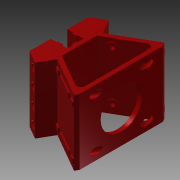
# Autodesk Inventor part: lower corner
Saved by Autodesk Inventor 2015 SP1 (Build 190203100, 203)
## iProperties
Created: 2015-01-28
Part Number: lower corner
Material: Generic
Document SubType Name: Modeling
Designer: Joseph
Density: 1 g/cm^3
Appearance: Red
Author: Joseph
Autodesk Inventor part; units mm, degrees
note: some values were not read from the file. Chosen so that the rebuilt part matches the saved one: direction of "Hole8".
sketch "Sketch1" plane through (0, 0, 0) normal (0, 0, 1) x (1, 0, 0)
  line L0 (7.9588, 40.9294) -> (17.9588, 23.6089)
  line L1 (17.9588, 23.6089) -> (65.5902, 51.1089)
  line L2 (7.9588, -48.8207) -> (17.9588, -31.5002)
  line L3 (17.9588, -31.5002) -> (65.5902, -59.0002)
  line L4 (65.5902, -59.0002) -> (68.0902, -54.6701)
  line L5 (65.5902, 51.1089) -> (68.0902, 46.7788)
  line L6 (17.039, 17.3044) -> (17.039, -25.1956)
  line L7 (-7.6578, 31.9131) -> (7.9588, 40.9294)
  line L8 (7.9588, -48.8207) -> (-7.6578, -39.8044)
  line L9 (63.0902, 43.892) -> (63.0902, -51.7833)
  line L10 (68.0902, 46.7788) -> (68.0902, -54.6701)
  line L11 (63.0902, 43.892) -> (17.039, 17.3044)
  line L12 (63.0902, -51.7833) -> (17.039, -25.1956)
  line L13 (63.0902, -12.2336) -> (68.0902, -12.2336) construction
  line L14 (63.0902, -51.7833) -> (60.5902, -56.1134) construction
  line L15 (63.0902, 43.892) -> (60.5902, 48.2222) construction
  line L16 (17.039, -3.9456) -> (63.0902, -3.9456) construction
  line L17 (-7.6578, 6.0639) -> (-7.6578, -13.9552) construction
  line L18 (-7.6578, 31.9131) -> (-7.6578, 6.0639)
  line L19 (-7.6578, -13.9552) -> (-7.6578, -39.8044)
  line L20 (-7.6578, -13.9552) -> (-0.4078, -13.9552)
  line L21 (5.0922, -13.9361) -> (12.3422, -13.9361)
  line L22 (12.3422, 6.0639) -> (5.0922, 6.0639)
  line L23 (-0.4078, 6.0639) -> (-7.6578, 6.0639)
  line L24 (12.3422, -6.6861) -> (10.8613, -6.6861)
  line L25 (10.8613, -6.6861) -> (10.8613, -1.1861)
  line L26 (10.8613, -1.1861) -> (12.3422, -1.1861)
  line L27 (5.0922, 6.0639) -> (5.0922, 4.5831)
  line L28 (5.0922, 4.5831) -> (-0.4078, 4.5831)
  line L29 (-0.4078, 4.5831) -> (-0.4078, 6.0639)
  line L30 (-0.4078, -13.9552) -> (-0.4078, -12.4552)
  line L31 (-0.4078, -12.4552) -> (5.0922, -12.4552)
  line L32 (5.0922, -12.4552) -> (5.0922, -13.9361)
  line L33 (12.3422, -13.9361) -> (12.3422, -6.6861)
  line L34 (12.3422, -1.1861) -> (12.3422, 6.0639)
  dimension "d11" = 20
  dimension "d12" = 55
  dimension "d110" = 42.5
  dimension "d176" = 5
  dimension "d177" = 60
  dimension "d178" = 120
  dimension "d179" = 60
  dimension "d181" = 20
  dimension "d184" = 1.5
  dimension "d185" = 5.5
  dimension "d186" = 20
  dimension "d195" = 34.8655
  dimension "d209" = 55
  constraints: 70 end point, 19 perpendicular, 15 equal length, 12 parallel, 6 point on line, 2 horizontal, 2 midpoint
  measures "d11" distance of L2.start L2.end
  measures "d12" distance of L2.end L3.end
  measures "d110" distance of L6.start L6.end
  measures "d176" distance of L3.end L4.end
  measures "d177" angle of L11 L12
  measures "d178" angle of L6 L12
  measures "d179" angle of L1 L3
  measures "d181" distance of L22.start L21.end
  measures "d184" distance of L20.end L30.end
  measures "d185" distance of L30.end L31.end
  measures "d186" distance between parallel lines of L17 L33
  measures "d195" distance from line of L0.start L22
  measures "d209" distance of L0.end L1.end
extrude "Extrusion13" add sketch "Sketch1" along normal blind 80
fillet "Fillet5" radius 5 2 edges at (63.0902, -51.7833, 40) (63.0902, 43.892, 40)
sketch "Sketch2" plane through (7.9588, 40.9294, 80) normal (0.8660254, 0.5, 0) x (0, 0, -1)
  line L0 (20, -20) -> (0, -20) construction
  circle A0 centre (10, -10) radius 10 construction
  circle A1 centre (70, -10) radius 10 construction
  line L1 (7, -21) -> (13, -21)
  line L2 (13, -21) -> (13, -19)
  line L3 (13, -19) -> (7, -19)
  line L4 (7, -19) -> (7, -21)
  line L5 (7, -21) -> (13, -19) construction
  line L6 (13, -21) -> (7, -19) construction
  line L7 (73, -21) -> (67, -21)
  line L8 (67, -21) -> (67, -19)
  line L9 (67, -19) -> (73, -19)
  line L10 (73, -19) -> (73, -21)
  line L11 (73, -21) -> (67, -19) construction
  line L12 (67, -21) -> (73, -19) construction
  line L13 (80, 0) -> (80, -20) projected
  line L14 (0, -20) -> (0, 0) projected
  line L15 (80, -20) -> (0, -20) projected
  line L16 (13, -19) -> (67, -19) construction
  point P0 (60, -34.2995)
  point P1 (10, -20)
  point P2 (70, -20)
  dimension "d11" = 20
  dimension "d168" = 20
  dimension "d19" = 20
  dimension "d23" = 6
  dimension "d24" = 2
  dimension "d25" = 6
  dimension "d26" = 2
  constraints: 28 end point, 5 horizontal, 4 midpoint, 4 parallel, 3 perpendicular, 2 vertical, 2 vertical alignment, 4 other
  measures "d19" distance of L0.start L0.end
  measures "d23" distance of L3.end L2.end
  measures "d24" distance of L2.end L1.end
  measures "d25" distance of L8.end L9.end
  measures "d26" distance of L7.end L8.end
extrude "Extrusion2" add sketch "Sketch2" along normal up to surface (55 mm away) from surface at 0
sketch "Sketch8" plane through (17.9588, -31.5002, 80) normal (0.8660254, -0.5, 0) x (0, 0, -1)
  line L0 (0, 0) -> (20, 0) construction
  line L1 (80, 0) -> (60, 0) construction
  line L2 (60, 0) -> (0, 0)
  line L3 (20, 0) -> (0, 0) construction
  line L4 (40, 0) -> (60, 0) construction
  line L5 (80, 0) -> (80, -20) projected
  circle A0 centre (70, -10) radius 10 construction
  line L6 (80, 0) -> (0, 0) projected
  line L7 (70, 0) -> (70, -20) construction
  line L8 (80, -20) -> (0, -20) construction
  line L9 (40, -20) -> (40, 0) construction
  line L10 (72.75, 1.5) -> (67.25, 1.5)
  line L11 (67.25, 1.5) -> (67.25, -1.5)
  line L12 (67.25, -1.5) -> (72.75, -1.5)
  line L13 (72.75, -1.5) -> (72.75, 1.5)
  line L14 (72.75, 1.5) -> (67.25, -1.5) construction
  line L15 (67.25, 1.5) -> (72.75, -1.5) construction
  line L16 (10, 0) -> (10, -20) construction
  line L17 (7.25, -1.5) -> (12.75, -1.5)
  line L18 (12.75, -1.5) -> (12.75, 1.5)
  line L19 (12.75, 1.5) -> (7.25, 1.5)
  line L20 (7.25, 1.5) -> (7.25, -1.5)
  line L21 (7.25, -1.5) -> (12.75, 1.5) construction
  line L22 (12.75, -1.5) -> (7.25, 1.5) construction
  point P0 (60, 16.0535)
  point P1 (60, 3.2816)
  dimension "d169" = 20
  dimension "d171" = 5.5
  dimension "d172" = 3
  dimension "d173" = 5.5
  dimension "d174" = 3
  constraints: 40 end point, 6 midpoint, 4 horizontal, 4 parallel, 2 perpendicular, 2 point on circle, 2 symmetric about line, 2 tangent, 1 centre point, 1 line through centre, 1 point on line, 1 vertical
  measures "d169" diameter of A0
  measures "d171" distance of L12.end L11.end
  measures "d172" distance of L11.end L10.end
  measures "d173" distance of L19.end L18.end
  measures "d174" distance of L18.end L17.end
extrude "Extrusion7" add sketch "Sketch8" along normal up to surface (55 mm away) from surface at 0
ref_plane "Work Plane20" through (33.539, 3.3832, 80) normal (0.5, 0.8660254, 0) x (0.8660254, -0.5, 0)
sketch "Sketch9" plane through (33.539, 3.3832, 80) normal (0.5, 0.8660254, 0) x (0.8660254, -0.5, 0)
  line L0 (58.9488, 70) -> (1.9893, 70) construction
  line L1 (48.9488, 10) -> (13.9488, 10) construction
  line L2 (13.9488, 10) -> (13.9488, 70) construction
  line L3 (13.9488, 70) -> (48.9488, 70) construction
  line L4 (48.9488, 70) -> (48.9488, 10) construction
  line L5 (58.9488, 72.75) -> (58.9488, 67.25) construction
  line L6 (58.9488, 12.75) -> (58.9488, 7.25) construction
  line L7 (48.9488, 10) -> (58.9488, 10) construction
  point P0 (-26.8584, -7)
  dimension "d73" = 35
  dimension "d205" = 10
  constraints: 12 end point, 4 coincident, 2 horizontal, 2 midpoint, 2 parallel, 1 collinear, 1 perpendicular, 1 point on line
  measures "d73" distance of L1.end L7.start
  measures "d205" distance of L7.start L7.end
hole "Hole2" at (75.93, -21.0912, 70) at (45.6191, -3.5912, 70) at (75.93, -21.0912, 10) at (45.6191, -3.5912, 10) direction (-0.5, -0.8660254, 0) diameter 4.5 end through all counterbore diameter 8 counterbore depth 32 clearance for "Socket Head Cap Screw" size "M4" standard "Ansi Metric M Profile"
ref_plane "Work Plane21" through (33.539, -11.2745, 0) normal (0.5, -0.8660254, 0) x (0.8660254, 0.5, 0)
sketch "Sketch10" plane through (33.539, -11.2745, 0) normal (0.5, -0.8660254, 0) x (0.8660254, 0.5, 0)
  line L0 (48.9488, 70) -> (13.9488, 70) construction
  line L1 (13.9488, 70) -> (13.9488, 10) construction
  line L2 (13.9488, 10) -> (48.9488, 10) construction
  line L3 (48.9488, 10) -> (48.9488, 70) construction
  line L4 (58.9488, 13) -> (58.9488, 7) construction
  line L5 (58.9488, 73) -> (58.9488, 67) construction
  line L6 (48.9488, 10) -> (58.9488, 10) construction
  line L7 (48.9488, 70) -> (58.9488, 70) construction
  point P0 (-25.1395, 13)
  dimension "d74" = 35
  dimension "d208" = 10
  constraints: 12 end point, 4 coincident, 2 collinear, 2 midpoint, 2 parallel, 1 horizontal, 1 perpendicular
  measures "d74" distance of L2.end L1.end
  measures "d208" distance between parallel lines of L3 L4
hole "Hole3" at (75.93, 13.1999, 70) at (75.93, 13.1999, 10) at (45.6191, -4.3001, 10) at (45.6191, -4.3001, 70) direction (-0.5, 0.8660254, 0) diameter 4.5 end through all counterbore diameter 8 counterbore depth 32 clearance for "Socket Head Cap Screw" size "M4" standard "Ansi Metric M Profile"
ref_plane "Work Plane18" through (7.9588, 40.9294, 0) normal (0, -1, 0) x (1, 0, 0)
sketch "Sketch20" plane through (7.9588, 40.9294, 0) normal (0, -1, 0) x (1, 0, 0)
  line L0 (-2.8667, 0) -> (-8.3667, 0) construction
  line L1 (-8.3667, 80) -> (-2.8667, 80) construction
  line L2 (-5.6167, 0) -> (-5.6167, 80) construction
  circle A0 centre (-5.6167, 70) radius 10
  circle A1 centre (-5.6167, 10) radius 10
  circle A2 centre (-5.6167, 40) radius 10
  point P0 (-7.9588, 0)
  point P1 (-5.6167, 30)
  point P2 (-5.6167, 50)
  dimension "d210" = 20
  dimension "d211" = 20
  dimension "d212" = 20
  constraints: 4 point on line, 3 centre point, 3 midpoint, 2 end point, 2 point on circle, 2 tangent
  measures "d210" diameter of A0
  measures "d211" diameter of A1
  measures "d212" diameter of A2
hole "Hole7" at (2.3422, 40.9294, 30) at (2.3422, 40.9294, 50) at (2.3422, 40.9294, 70) at (2.3422, 40.9294, 10) direction (0, -1, 0) diameter 4.5 end up to surface counterbore diameter 8 counterbore depth 16.35 clearance for "Socket Head Cap Screw" size "M4" standard "Ansi Metric M Profile"
ref_plane "Work Plane19" through (7.9588, -48.8207, 0) normal (0, -1, 0) x (1, 0, 0)
sketch "Sketch21" plane through (7.9588, -48.8207, 0) normal (0, -1, 0) x (1, 0, 0)
  line L0 (-8.3667, 0) -> (-2.8667, 0) projected
  line L1 (-2.8667, 80) -> (-8.3667, 80) projected
  line L2 (-5.6167, 80) -> (-5.6167, 0) construction
  circle A0 centre (-5.6167, 40) radius 10 construction
  circle A1 centre (-5.6167, 10) radius 10
  circle A2 centre (-5.6167, 70) radius 10
  point P0 (-7.9588, 0)
  point P1 (-5.6167, 50)
  point P2 (-5.6167, 30)
  point P3 (-5.6167, 70.2671)
  dimension "d196" = 20
  dimension "d213" = 20
  dimension "d214" = 20
  constraints: 4 point on line, 3 centre point, 3 midpoint, 2 end point, 2 point on circle, 2 tangent, 1 coincident
  measures "d196" diameter of A0
  measures "d213" diameter of A1
  measures "d214" diameter of A2
hole "Hole8" at (2.3422, -48.8207, 50) at (2.3422, -48.8207, 30) at (2.3422, -48.8207, 70.2671) at (2.3422, -48.8207, 10) direction (0, 1, 0) diameter 4.5 end up to surface counterbore diameter 8 counterbore depth 16.35 clearance for "Socket Head Cap Screw" size "M4" standard "Ansi Metric M Profile"
sketch "Sketch22" plane through (68.0902, -54.6701, 0) normal (1, 0, 0) x (0, 0, -1)
  circle A0 centre (-40, 50.7244) radius 25
  point P0 (0, 54.6701)
  dimension "d215" = 50
  constraints: 1 centre point
  measures "d215" diameter of A0
extrude "Extrusion14" cut sketch "Sketch22" against normal up to surface (5 mm away)
sketch "Sketch23" plane through (17.039, -25.1956, 0) normal (1, 0, 0) x (0, 0, -1)
  line L0 (0, 42.5) -> (0, 0) projected
  circle A0 centre (0, 21.25) radius 7.5
  point P0 (0, 25.1956)
  dimension "d218" = 15
  constraints: 1 centre point, 1 midpoint
  measures "d218" diameter of A0
extrude "Extrusion15" cut sketch "Sketch23" against normal up to surface (6.1777 mm away)
fillet "Fillet6" radius 2 4 edges at (17.039, -25.1956, 40) (17.039, 17.3044, 40) (68.0902, -54.6701, 40) (68.0902, 46.7788, 40)
sketch "Sketch24" plane through (55.5902, 39.5619, 0) normal (0.5, -0.8660254, 0) x (0.8660254, 0.5, 0)
  circle A0 centre (-30.5662, 70) radius 2.25 projected
  circle A1 centre (-30.5662, 10) radius 2.25 projected
  circle A2 centre (-30.5662, 70) radius 6
  circle A3 centre (-30.5662, 10) radius 6
  circle A4 centre (4.4338, 70) radius 2.25 projected
  circle A5 centre (4.4338, 10) radius 2.25 projected
  circle A6 centre (4.4338, 70) radius 6
  circle A7 centre (4.4338, 10) radius 6
  point P0 (-67.9235, 0)
  dimension "d222" = 12
  dimension "d223" = 12
  dimension "d228" = 12
  dimension "d229" = 12
  constraints: 4 centre point, 4 coincident
  measures "d222" diameter of A2
  measures "d223" diameter of A3
  measures "d228" diameter of A6
  measures "d229" diameter of A7
extrude "Extrusion16" add sketch "Sketch24" along normal blind 1
sketch "Sketch26" plane through (55.5902, -47.4532, 80) normal (0.5, 0.8660254, 0) x (0.8660254, -0.5, 0)
  circle A0 centre (-30.5662, 10) radius 2.25 projected
  circle A1 centre (-30.5662, 70) radius 2.25 projected
  circle A2 centre (4.4338, 10) radius 2.25 projected
  circle A3 centre (4.4338, 70) radius 2.25 projected
  circle A4 centre (-30.5662, 10) radius 6
  circle A5 centre (-30.5662, 70) radius 6
  circle A6 centre (4.4338, 70) radius 6
  circle A7 centre (4.4338, 10) radius 6
  point P0 (-71.8691, 80)
  dimension "d230" = 12
  dimension "d231" = 12
  dimension "d232" = 12
  dimension "d233" = 12
  constraints: 4 centre point, 4 coincident
  measures "d230" diameter of A4
  measures "d231" diameter of A5
  measures "d232" diameter of A6
  measures "d233" diameter of A7
extrude "Extrusion17" add sketch "Sketch26" along normal blind 1
sketch "Sketch27" plane through (17.2088, -32.7992, 67.25) normal (-0.5, -0.8660254, 0) x (0.8660254, -0.5, 0)
  circle A0 centre (45, 2.75) radius 2.25 projected
  circle A1 centre (10, 2.75) radius 2.25 projected
  circle A2 centre (10, -57.25) radius 2.25 projected
  circle A3 centre (45, -57.25) radius 2.25 projected
  line L0 (6.875, -60.375) -> (13.125, -60.375)
  line L1 (13.125, -60.375) -> (13.125, -54.125)
  line L2 (13.125, -54.125) -> (6.875, -54.125)
  line L3 (6.875, -54.125) -> (6.875, -60.375)
  line L4 (6.875, -60.375) -> (13.125, -54.125) construction
  line L5 (13.125, -60.375) -> (6.875, -54.125) construction
  line L6 (41.875, -60.375) -> (48.125, -60.375)
  line L7 (48.125, -60.375) -> (48.125, -54.125)
  line L8 (48.125, -54.125) -> (41.875, -54.125)
  line L9 (41.875, -54.125) -> (41.875, -60.375)
  line L10 (41.875, -60.375) -> (48.125, -54.125) construction
  line L11 (48.125, -60.375) -> (41.875, -54.125) construction
  line L12 (41.875, -0.375) -> (48.125, -0.375)
  line L13 (48.125, -0.375) -> (48.125, 5.875)
  line L14 (48.125, 5.875) -> (41.875, 5.875)
  line L15 (41.875, 5.875) -> (41.875, -0.375)
  line L16 (41.875, -0.375) -> (48.125, 5.875) construction
  line L17 (48.125, -0.375) -> (41.875, 5.875) construction
  line L18 (6.875, -0.375) -> (13.125, -0.375)
  line L19 (13.125, -0.375) -> (13.125, 5.875)
  line L20 (13.125, 5.875) -> (6.875, 5.875)
  line L21 (6.875, 5.875) -> (6.875, -0.375)
  line L22 (6.875, -0.375) -> (13.125, 5.875) construction
  line L23 (13.125, -0.375) -> (6.875, 5.875) construction
  point P0 (-31.3029, -67.25)
  dimension "d236" = 6.25
  dimension "d237" = 6.25
  dimension "d238" = 6.25
  dimension "d239" = 6.25
  dimension "d240" = 6.25
  dimension "d241" = 6.25
  dimension "d242" = 6.25
  dimension "d243" = 6.25
  constraints: 48 end point, 8 midpoint, 8 parallel, 4 horizontal, 4 perpendicular
  measures "d236" distance of L2.end L1.end
  measures "d237" distance of L1.end L0.end
  measures "d238" distance of L8.end L7.end
  measures "d239" distance of L7.end L6.end
  measures "d240" distance of L14.end L13.end
  measures "d241" distance of L13.end L12.end
  measures "d242" distance of L20.end L19.end
  measures "d243" distance of L19.end L18.end
extrude "Extrusion18" cut sketch "Sketch27" against normal up to surface (1.5 mm away)
sketch "Sketch28" plane through (17.4588, 24.4749, 73) normal (-0.5, 0.8660254, 0) x (0.8660254, 0.5, 0)
  circle A0 centre (45, 3) radius 2.25 projected
  circle A1 centre (10, 3) radius 2.25 projected
  circle A2 centre (10, 63) radius 2.25 projected
  circle A3 centre (45, 63) radius 2.25 projected
  line L0 (6.875, -0.125) -> (13.125, -0.125)
  line L1 (13.125, -0.125) -> (13.125, 6.125)
  line L2 (13.125, 6.125) -> (6.875, 6.125)
  line L3 (6.875, 6.125) -> (6.875, -0.125)
  line L4 (6.875, -0.125) -> (13.125, 6.125) construction
  line L5 (13.125, -0.125) -> (6.875, 6.125) construction
  line L6 (41.875, -0.125) -> (48.125, -0.125)
  line L7 (48.125, -0.125) -> (48.125, 6.125)
  line L8 (48.125, 6.125) -> (41.875, 6.125)
  line L9 (41.875, 6.125) -> (41.875, -0.125)
  line L10 (41.875, -0.125) -> (48.125, 6.125) construction
  line L11 (48.125, -0.125) -> (41.875, 6.125) construction
  line L12 (41.875, 59.875) -> (48.125, 59.875)
  line L13 (48.125, 59.875) -> (48.125, 66.125)
  line L14 (48.125, 66.125) -> (41.875, 66.125)
  line L15 (41.875, 66.125) -> (41.875, 59.875)
  line L16 (41.875, 59.875) -> (48.125, 66.125) construction
  line L17 (48.125, 59.875) -> (41.875, 66.125) construction
  line L18 (6.875, 59.875) -> (13.125, 59.875)
  line L19 (13.125, 59.875) -> (13.125, 66.125)
  line L20 (13.125, 66.125) -> (6.875, 66.125)
  line L21 (6.875, 66.125) -> (6.875, 59.875)
  line L22 (6.875, 59.875) -> (13.125, 66.125) construction
  line L23 (13.125, 59.875) -> (6.875, 66.125) construction
  point P0 (-27.3573, 73)
  dimension "d246" = 6.25
  dimension "d247" = 6.25
  dimension "d248" = 6.25
  dimension "d249" = 6.25
  dimension "d250" = 6.25
  dimension "d251" = 6.25
  dimension "d252" = 6.25
  dimension "d253" = 6.25
  constraints: 48 end point, 8 midpoint, 8 parallel, 4 horizontal, 4 perpendicular
  measures "d246" distance of L2.end L1.end
  measures "d247" distance of L1.end L0.end
  measures "d248" distance of L8.end L7.end
  measures "d249" distance of L7.end L6.end
  measures "d250" distance of L14.end L13.end
  measures "d251" distance of L13.end L12.end
  measures "d252" distance of L20.end L19.end
  measures "d253" distance of L19.end L18.end
extrude "Extrusion19" cut sketch "Sketch28" against normal up to surface (1 mm away)
sketch "Sketch29" plane through (-0.4078, -12.4552, 0) normal (0, 1, 0) x (1, 0, 0)
  circle A0 centre (2.75, -70.2671) radius 2.25 projected
  circle A1 centre (2.75, -50) radius 2.25 projected
  circle A2 centre (2.75, -30) radius 2.25 projected
  circle A3 centre (2.75, -10) radius 2.25 projected
  line L0 (-0.375, -73.3921) -> (5.875, -73.3921)
  line L1 (5.875, -73.3921) -> (5.875, -67.1421)
  line L2 (5.875, -67.1421) -> (-0.375, -67.1421)
  line L3 (-0.375, -67.1421) -> (-0.375, -73.3921)
  line L4 (-0.375, -73.3921) -> (5.875, -67.1421) construction
  line L5 (5.875, -73.3921) -> (-0.375, -67.1421) construction
  line L6 (-0.375, -53.125) -> (5.875, -53.125)
  line L7 (5.875, -53.125) -> (5.875, -46.875)
  line L8 (5.875, -46.875) -> (-0.375, -46.875)
  line L9 (-0.375, -46.875) -> (-0.375, -53.125)
  line L10 (-0.375, -53.125) -> (5.875, -46.875) construction
  line L11 (5.875, -53.125) -> (-0.375, -46.875) construction
  line L12 (-0.375, -33.125) -> (5.875, -33.125)
  line L13 (5.875, -33.125) -> (5.875, -26.875)
  line L14 (5.875, -26.875) -> (-0.375, -26.875)
  line L15 (-0.375, -26.875) -> (-0.375, -33.125)
  line L16 (-0.375, -33.125) -> (5.875, -26.875) construction
  line L17 (5.875, -33.125) -> (-0.375, -26.875) construction
  line L18 (-0.375, -13.125) -> (5.875, -13.125)
  line L19 (5.875, -13.125) -> (5.875, -6.875)
  line L20 (5.875, -6.875) -> (-0.375, -6.875)
  line L21 (-0.375, -6.875) -> (-0.375, -13.125)
  line L22 (-0.375, -13.125) -> (5.875, -6.875) construction
  line L23 (5.875, -13.125) -> (-0.375, -6.875) construction
  point P0 (0.4078, 0)
  dimension "d256" = 6.25
  dimension "d257" = 6.25
  dimension "d258" = 6.25
  dimension "d259" = 6.25
  dimension "d260" = 6.25
  dimension "d261" = 6.25
  dimension "d262" = 6.25
  dimension "d263" = 6.25
  constraints: 48 end point, 8 midpoint, 8 parallel, 4 horizontal, 4 perpendicular
  measures "d256" distance of L2.end L1.end
  measures "d257" distance of L1.end L0.end
  measures "d258" distance of L8.end L7.end
  measures "d259" distance of L7.end L6.end
  measures "d260" distance of L14.end L13.end
  measures "d261" distance of L13.end L12.end
  measures "d262" distance of L20.end L19.end
  measures "d263" distance of L19.end L18.end
extrude "Extrusion20" cut sketch "Sketch29" against normal up to surface (1.5 mm away)
sketch "Sketch30" plane through (-0.4078, 4.5831, 0) normal (0, -1, 0) x (1, 0, 0)
  circle A0 centre (2.75, 10) radius 2.25 projected
  circle A1 centre (2.75, 50) radius 2.25 projected
  circle A2 centre (2.75, 30) radius 2.25 projected
  circle A3 centre (2.75, 70) radius 2.25 projected
  line L0 (5.875, 6.875) -> (-0.375, 6.875)
  line L1 (-0.375, 6.875) -> (-0.375, 13.125)
  line L2 (-0.375, 13.125) -> (5.875, 13.125)
  line L3 (5.875, 13.125) -> (5.875, 6.875)
  line L4 (5.875, 6.875) -> (-0.375, 13.125) construction
  line L5 (-0.375, 6.875) -> (5.875, 13.125) construction
  line L6 (5.875, 26.875) -> (-0.375, 26.875)
  line L7 (-0.375, 26.875) -> (-0.375, 33.125)
  line L8 (-0.375, 33.125) -> (5.875, 33.125)
  line L9 (5.875, 33.125) -> (5.875, 26.875)
  line L10 (5.875, 26.875) -> (-0.375, 33.125) construction
  line L11 (-0.375, 26.875) -> (5.875, 33.125) construction
  line L12 (5.875, 46.875) -> (-0.375, 46.875)
  line L13 (-0.375, 46.875) -> (-0.375, 53.125)
  line L14 (-0.375, 53.125) -> (5.875, 53.125)
  line L15 (5.875, 53.125) -> (5.875, 46.875)
  line L16 (5.875, 46.875) -> (-0.375, 53.125) construction
  line L17 (-0.375, 46.875) -> (5.875, 53.125) construction
  line L18 (5.875, 66.875) -> (-0.375, 66.875)
  line L19 (-0.375, 66.875) -> (-0.375, 73.125)
  line L20 (-0.375, 73.125) -> (5.875, 73.125)
  line L21 (5.875, 73.125) -> (5.875, 66.875)
  line L22 (5.875, 66.875) -> (-0.375, 73.125) construction
  line L23 (-0.375, 66.875) -> (5.875, 73.125) construction
  point P0 (0.4078, 0)
  dimension "d266" = 6.25
  dimension "d267" = 6.25
  dimension "d268" = 6.25
  dimension "d269" = 6.25
  dimension "d270" = 6.25
  dimension "d271" = 6.25
  dimension "d272" = 6.25
  dimension "d273" = 6.25
  constraints: 48 end point, 8 midpoint, 8 parallel, 4 horizontal, 4 perpendicular
  measures "d266" distance of L1.end L2.end
  measures "d267" distance of L0.end L1.end
  measures "d268" distance of L7.end L8.end
  measures "d269" distance of L6.end L7.end
  measures "d270" distance of L13.end L14.end
  measures "d271" distance of L12.end L13.end
  measures "d272" distance of L19.end L20.end
  measures "d273" distance of L18.end L19.end
extrude "Extrusion21" cut sketch "Sketch30" against normal up to surface (1.4809 mm away)
body "Solid1"
body "Solid2"
